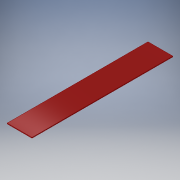
# Autodesk Inventor part: Drive Base Cover
Saved by Autodesk Inventor 2019.4 (Build 234330000, 330)
## iProperties
Created: 2020-01-23
Part Number: Drive Base Cover
Material: Polycarbonate, Smoke
Document SubType Name: Modeling
Designer: admin
Density: 1.2 g/cm^3
Appearance: Red
Author: admin
Autodesk Inventor part; units mm, degrees
ref_plane "YZ Plane" through (0, 0, 0) normal (1, 0, 0) x (0, 1, 0)
ref_plane "XZ Plane" through (0, 0, 0) normal (0, 1, 0) x (-1, 0, 0)
ref_plane "XY Plane" through (0, 0, 0) normal (0, 0, 1) x (1, 0, 0)
sketch "Sketch1" plane through (0, 0, 0) normal (0, 1, 0) x (-1, 0, 0)
  line L0 (-82, 465) -> (82, 465)
  line L1 (82, 465) -> (82, -465)
  line L2 (82, -465) -> (-82, -465)
  line L3 (-82, -465) -> (-82, 465)
  line L4 (-82, 465) -> (82, -465) construction
  line L5 (82, 465) -> (-82, -465) construction
  point P0 (0, 0)
  dimension "d0" = 930
  dimension "d1" = 164
  constraints: 12 end point, 2 midpoint, 2 parallel, 1 horizontal, 1 perpendicular
  measures "d0" distance of L0.end L1.end
  measures "d1" distance of L1.end L2.end
extrude "Extrusion1" add sketch "Sketch1" along normal mid plane 5
body "Solid1"
